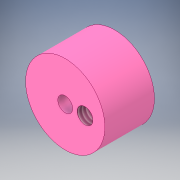
# Autodesk Inventor part: MotorArm
Saved by Autodesk Inventor 2017 (Build 210142000, 142)
## iProperties
Created: 2017-02-08
Part Number: MotorArm
Material: Aluminum 6061
Document SubType Name: Modeling
Designer: Joseph
Density: 2.7 g/cm^3
Appearance: Pink
Author: Joseph
Autodesk Inventor part; units mm, degrees
ref_plane "YZ Plane" through (0, 0, 0) normal (1, 0, 0) x (0, 1, 0)
ref_plane "XZ Plane" through (0, 0, 0) normal (0, 1, 0) x (-1, 0, 0)
ref_plane "XY Plane" through (0, 0, 0) normal (0, 0, 1) x (1, 0, 0)
sketch "Sketch1" plane through (0, 0, 0) normal (0, 0, 1) x (1, 0, 0)
  circle A0 centre (0, 0) radius 4
  dimension "d0" = 8
  constraints: 1 centre point, 1 coincident
  measures "d0" diameter of A0
extrude "Extrusion1" add sketch "Sketch1" along normal blind 5
sketch "Sketch2" plane through (0, 0, 5) normal (0, 0, 1) x (1, 0, 0)
  circle A0 centre (0, 0) radius 0.75
  dimension "d3" = 1.5
  constraints: 1 centre point, 1 coincident
  measures "d3" diameter of A0
extrude "Extrusion2" cut sketch "Sketch2" against normal blind 5
sketch "Sketch3" plane through (0, 0, 5) normal (0, 0, 1) x (1, 0, 0)
  circle A0 centre (2, 0) radius 0.8
  point P0 (0, 0)
  dimension "d6" = 1.6
  dimension "d7" = 0
  dimension "d8" = 2
  constraints: 1 centre point
  measures "d6" diameter of A0
  measures "d7" vertical distance of A0.centre point (0, 0)
  measures "d8" distance of point (0, 0) A0.centre
extrude "Extrusion3" cut sketch "Sketch3" against normal blind 5
thread "Thread1" size "M2x0.4" class "6H" standard "ANSI Metric M Profile" full length
body "Solid1"
